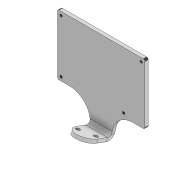
# Autodesk Inventor part: HMI achterzijde
Saved by Autodesk Inventor 2020.3 (Build 243373000, 373)
## iProperties
Created: 2020-12-03
Part Number: HMI achterzijde
Material: Generic
Document SubType Name: Sheet Metal
Designer: Svend
Density: 1 g/cm^3
Sheet Metal Rule: Default_mm
Appearance: Default
Flat Pattern Width: 13.0658 cm
Flat Pattern Length: 10.4848 cm
Flat Pattern Area: 136.992 cm^2
Sheet Metal Width: 130,658 mm
Sheet Metal Length: 104,848 mm
Sheet Metal Area: 13699,236 mm^2
Author: Svend
Autodesk Inventor part; units mm, degrees
ref_plane "YZ Plane" through (0, 0, 0) normal (1, 0, 0) x (0, 1, 0)
ref_plane "XZ Plane" through (0, 0, 0) normal (0, 1, 0) x (-1, 0, 0)
ref_plane "XY Plane" through (0, 0, 0) normal (0, 0, 1) x (1, 0, 0)
ref_plane "Work Plane1" through (0, 0, 0) normal (0, 0, 1) x (1, 0, 0)
sketch "Sketch1" plane through (0, 0, 0) normal (0, 0, 1) x (1, 0, 0)
  line L0 (-22.2591, 4.439) -> (-22.2701, 4.6145)
  line L1 (-22.2701, 4.2636) -> (-22.2591, 4.439)
  line L2 (-22.2701, 4.2636) -> (-22.3031, 4.0909)
  line L3 (-22.3574, 3.9237) -> (-22.3031, 4.0909)
  line L4 (-22.4322, 3.7646) -> (-22.3574, 3.9237)
  line L5 (-22.5265, 3.6161) -> (-22.4322, 3.7646)
  line L6 (-22.6385, 3.4807) -> (-22.5265, 3.6161)
  line L7 (-22.7667, 3.3603) -> (-22.6385, 3.4807)
  line L8 (-22.9089, 3.257) -> (-22.7667, 3.3603)
  line L9 (-23.063, 3.1723) -> (-22.9089, 3.257)
  line L10 (-23.2265, 3.1076) -> (-23.063, 3.1723)
  line L11 (-23.3967, 3.0638) -> (-23.2265, 3.1076)
  line L12 (-23.5712, 3.0418) -> (-23.3967, 3.0638)
  line L13 (-23.747, 3.0418) -> (-23.5712, 3.0418)
  line L14 (-23.9214, 3.0638) -> (-23.747, 3.0418)
  line L15 (-24.0917, 3.1076) -> (-23.9214, 3.0638)
  line L16 (-24.2552, 3.1723) -> (-24.0917, 3.1076)
  line L17 (-24.4092, 3.257) -> (-24.2552, 3.1723)
  line L18 (-24.5515, 3.3603) -> (-24.4092, 3.257)
  line L19 (-24.6796, 3.4807) -> (-24.5515, 3.3603)
  line L20 (-24.7917, 3.6161) -> (-24.6796, 3.4807)
  line L21 (-24.8859, 3.7646) -> (-24.7917, 3.6161)
  line L22 (-24.9608, 3.9237) -> (-24.8859, 3.7646)
  line L23 (-25.0151, 4.0909) -> (-24.9608, 3.9237)
  line L24 (-25.048, 4.2636) -> (-25.0151, 4.0909)
  line L25 (-25.0591, 4.439) -> (-25.048, 4.2636)
  line L26 (-25.048, 4.6145) -> (-25.0591, 4.439)
  line L27 (-25.0151, 4.7872) -> (-25.048, 4.6145)
  line L28 (-24.9608, 4.9544) -> (-25.0151, 4.7872)
  line L29 (-24.8859, 5.1135) -> (-24.9608, 4.9544)
  line L30 (-24.7917, 5.2619) -> (-24.8859, 5.1135)
  line L31 (-24.6796, 5.3974) -> (-24.7917, 5.2619)
  line L32 (-24.5515, 5.5178) -> (-24.6796, 5.3974)
  line L33 (-24.4092, 5.6211) -> (-24.5515, 5.5178)
  line L34 (-24.2552, 5.7058) -> (-24.4092, 5.6211)
  line L35 (-24.0917, 5.7705) -> (-24.2552, 5.7058)
  line L36 (-23.9214, 5.8142) -> (-24.0917, 5.7705)
  line L37 (-23.747, 5.8363) -> (-23.9214, 5.8142)
  line L38 (-23.5712, 5.8363) -> (-23.747, 5.8363)
  line L39 (-23.3967, 5.8142) -> (-23.5712, 5.8363)
  line L40 (-23.2265, 5.7705) -> (-23.3967, 5.8142)
  line L41 (-23.063, 5.7058) -> (-23.2265, 5.7705)
  line L42 (-22.9089, 5.6211) -> (-23.063, 5.7058)
  line L43 (-22.7667, 5.5178) -> (-22.9089, 5.6211)
  line L44 (-22.6385, 5.3974) -> (-22.7667, 5.5178)
  line L45 (-22.5265, 5.2619) -> (-22.6385, 5.3974)
  line L46 (-22.4322, 5.1135) -> (-22.5265, 5.2619)
  line L47 (-22.3574, 4.9544) -> (-22.4322, 5.1135)
  line L48 (-22.3031, 4.7872) -> (-22.3574, 4.9544)
  line L49 (-22.2701, 4.6145) -> (-22.3031, 4.7872)
  line L50 (-1.2701, 68.1645) -> (-1.3031, 68.3372)
  line L51 (-1.2591, 67.989) -> (-1.2701, 68.1645)
  line L52 (-1.2701, 67.8135) -> (-1.2591, 67.989)
  line L53 (-1.2701, 67.8135) -> (-1.3031, 67.6408)
  line L54 (-1.3574, 67.4736) -> (-1.3031, 67.6408)
  line L55 (-1.4323, 67.3145) -> (-1.3574, 67.4736)
  line L56 (-1.5265, 67.1661) -> (-1.4323, 67.3145)
  line L57 (-1.6385, 67.0306) -> (-1.5265, 67.1661)
  line L58 (-1.7667, 66.9103) -> (-1.6385, 67.0306)
  line L59 (-1.9089, 66.8069) -> (-1.7667, 66.9103)
  line L60 (-2.063, 66.7222) -> (-1.9089, 66.8069)
  line L61 (-2.2265, 66.6576) -> (-2.063, 66.7222)
  line L62 (-2.3967, 66.6138) -> (-2.2265, 66.6576)
  line L63 (-2.5712, 66.5918) -> (-2.3967, 66.6138)
  line L64 (-2.747, 66.5918) -> (-2.5712, 66.5918)
  line L65 (-2.9214, 66.6138) -> (-2.747, 66.5918)
  line L66 (-3.0917, 66.6576) -> (-2.9214, 66.6138)
  line L67 (-3.2552, 66.7222) -> (-3.0917, 66.6576)
  line L68 (-3.4092, 66.8069) -> (-3.2552, 66.7222)
  line L69 (-3.5515, 66.9103) -> (-3.4092, 66.8069)
  line L70 (-3.6796, 67.0306) -> (-3.5515, 66.9103)
  line L71 (-3.7917, 67.1661) -> (-3.6796, 67.0306)
  line L72 (-3.8859, 67.3145) -> (-3.7917, 67.1661)
  line L73 (-3.9608, 67.4736) -> (-3.8859, 67.3145)
  line L74 (-4.0151, 67.6408) -> (-3.9608, 67.4736)
  line L75 (-4.048, 67.8135) -> (-4.0151, 67.6408)
  line L76 (-4.0591, 67.989) -> (-4.048, 67.8135)
  line L77 (-4.048, 68.1645) -> (-4.0591, 67.989)
  line L78 (-4.0151, 68.3372) -> (-4.048, 68.1645)
  line L79 (-3.9608, 68.5044) -> (-4.0151, 68.3372)
  line L80 (-3.8859, 68.6635) -> (-3.9608, 68.5044)
  line L81 (-3.7917, 68.8119) -> (-3.8859, 68.6635)
  line L82 (-3.6796, 68.9474) -> (-3.7917, 68.8119)
  line L83 (-3.5515, 69.0677) -> (-3.6796, 68.9474)
  line L84 (-3.4092, 69.1711) -> (-3.5515, 69.0677)
  line L85 (-3.2552, 69.2558) -> (-3.4092, 69.1711)
  line L86 (-3.0917, 69.3205) -> (-3.2552, 69.2558)
  line L87 (-2.9214, 69.3642) -> (-3.0917, 69.3205)
  line L88 (-2.747, 69.3862) -> (-2.9214, 69.3642)
  line L89 (-2.5712, 69.3862) -> (-2.747, 69.3862)
  line L90 (-2.3967, 69.3642) -> (-2.5712, 69.3862)
  line L91 (-2.2265, 69.3205) -> (-2.3967, 69.3642)
  line L92 (-2.063, 69.2558) -> (-2.2265, 69.3205)
  line L93 (-1.9089, 69.1711) -> (-2.063, 69.2558)
  line L94 (-1.7667, 69.0677) -> (-1.9089, 69.1711)
  line L95 (-1.6385, 68.9474) -> (-1.7667, 69.0677)
  line L96 (-1.5265, 68.8119) -> (-1.6385, 68.9474)
  line L97 (-1.4323, 68.6635) -> (-1.5265, 68.8119)
  line L98 (-1.3574, 68.5044) -> (-1.4323, 68.6635)
  line L99 (-1.3031, 68.3372) -> (-1.3574, 68.5044)
  line L100 (-99.0397, 69.3205) -> (-99.2032, 69.2558)
  line L101 (-98.8694, 69.3642) -> (-99.0397, 69.3205)
  line L102 (-98.695, 69.3862) -> (-98.8694, 69.3642)
  line L103 (-98.5192, 69.3862) -> (-98.695, 69.3862)
  line L104 (-98.3448, 69.3642) -> (-98.5192, 69.3862)
  line L105 (-98.1745, 69.3205) -> (-98.3448, 69.3642)
  line L106 (-98.011, 69.2558) -> (-98.1745, 69.3205)
  line L107 (-97.8569, 69.1711) -> (-98.011, 69.2558)
  line L108 (-97.7147, 69.0677) -> (-97.8569, 69.1711)
  line L109 (-97.5865, 68.9474) -> (-97.7147, 69.0677)
  line L110 (-97.4745, 68.8119) -> (-97.5865, 68.9474)
  line L111 (-97.3803, 68.6635) -> (-97.4745, 68.8119)
  line L112 (-97.3054, 68.5044) -> (-97.3803, 68.6635)
  line L113 (-97.2511, 68.3372) -> (-97.3054, 68.5044)
  line L114 (-97.2181, 68.1645) -> (-97.2511, 68.3372)
  line L115 (-97.2071, 67.989) -> (-97.2181, 68.1645)
  line L116 (-97.2181, 67.8135) -> (-97.2071, 67.989)
  line L117 (-97.2181, 67.8135) -> (-97.2511, 67.6408)
  line L118 (-97.3054, 67.4736) -> (-97.2511, 67.6408)
  line L119 (-97.3803, 67.3145) -> (-97.3054, 67.4736)
  line L120 (-97.4745, 67.1661) -> (-97.3803, 67.3145)
  line L121 (-97.5865, 67.0306) -> (-97.4745, 67.1661)
  line L122 (-97.7147, 66.9103) -> (-97.5865, 67.0306)
  line L123 (-97.8569, 66.8069) -> (-97.7147, 66.9103)
  line L124 (-98.011, 66.7222) -> (-97.8569, 66.8069)
  line L125 (-98.1745, 66.6576) -> (-98.011, 66.7222)
  line L126 (-98.3448, 66.6138) -> (-98.1745, 66.6576)
  line L127 (-98.5192, 66.5918) -> (-98.3448, 66.6138)
  line L128 (-98.695, 66.5918) -> (-98.5192, 66.5918)
  line L129 (-98.8694, 66.6138) -> (-98.695, 66.5918)
  line L130 (-99.0397, 66.6576) -> (-98.8694, 66.6138)
  line L131 (-99.2032, 66.7222) -> (-99.0397, 66.6576)
  line L132 (-99.3573, 66.8069) -> (-99.2032, 66.7222)
  line L133 (-99.4995, 66.9103) -> (-99.3573, 66.8069)
  line L134 (-99.6277, 67.0306) -> (-99.4995, 66.9103)
  line L135 (-99.7397, 67.1661) -> (-99.6277, 67.0306)
  line L136 (-99.8339, 67.3145) -> (-99.7397, 67.1661)
  line L137 (-99.9088, 67.4736) -> (-99.8339, 67.3145)
  line L138 (-99.9631, 67.6408) -> (-99.9088, 67.4736)
  line L139 (-99.9961, 67.8135) -> (-99.9631, 67.6408)
  line L140 (-100.0071, 67.989) -> (-99.9961, 67.8135)
  line L141 (-99.9961, 68.1645) -> (-100.0071, 67.989)
  line L142 (-99.9631, 68.3372) -> (-99.9961, 68.1645)
  line L143 (-99.9088, 68.5044) -> (-99.9631, 68.3372)
  line L144 (-99.8339, 68.6635) -> (-99.9088, 68.5044)
  line L145 (-99.7397, 68.8119) -> (-99.8339, 68.6635)
  line L146 (-99.6277, 68.9474) -> (-99.7397, 68.8119)
  line L147 (-99.4995, 69.0677) -> (-99.6277, 68.9474)
  line L148 (-99.3573, 69.1711) -> (-99.4995, 69.0677)
  line L149 (-99.2032, 69.2558) -> (-99.3573, 69.1711)
  line L150 (-99.3573, 3.257) -> (-99.2032, 3.1723)
  line L151 (-99.4995, 3.3603) -> (-99.3573, 3.257)
  line L152 (-99.6277, 3.4807) -> (-99.4995, 3.3603)
  line L153 (-99.7397, 3.6161) -> (-99.6277, 3.4807)
  line L154 (-99.8339, 3.7646) -> (-99.7397, 3.6161)
  line L155 (-99.9088, 3.9237) -> (-99.8339, 3.7646)
  line L156 (-99.9631, 4.0909) -> (-99.9088, 3.9237)
  line L157 (-99.9961, 4.2636) -> (-99.9631, 4.0909)
  line L158 (-100.0071, 4.439) -> (-99.9961, 4.2636)
  line L159 (-99.9961, 4.6145) -> (-100.0071, 4.439)
  line L160 (-99.9631, 4.7872) -> (-99.9961, 4.6145)
  line L161 (-99.9088, 4.9544) -> (-99.9631, 4.7872)
  line L162 (-99.8339, 5.1135) -> (-99.9088, 4.9544)
  line L163 (-99.7397, 5.2619) -> (-99.8339, 5.1135)
  line L164 (-99.6277, 5.3974) -> (-99.7397, 5.2619)
  line L165 (-99.4995, 5.5178) -> (-99.6277, 5.3974)
  line L166 (-99.3573, 5.6211) -> (-99.4995, 5.5178)
  line L167 (-99.2032, 5.7058) -> (-99.3573, 5.6211)
  line L168 (-99.0397, 5.7705) -> (-99.2032, 5.7058)
  line L169 (-98.8694, 5.8142) -> (-99.0397, 5.7705)
  line L170 (-98.695, 5.8363) -> (-98.8694, 5.8142)
  line L171 (-98.5192, 5.8363) -> (-98.695, 5.8363)
  line L172 (-98.3448, 5.8142) -> (-98.5192, 5.8363)
  line L173 (-98.1745, 5.7705) -> (-98.3448, 5.8142)
  line L174 (-98.011, 5.7058) -> (-98.1745, 5.7705)
  line L175 (-97.8569, 5.6211) -> (-98.011, 5.7058)
  line L176 (-97.7147, 5.5178) -> (-97.8569, 5.6211)
  line L177 (-97.5865, 5.3974) -> (-97.7147, 5.5178)
  line L178 (-97.4745, 5.2619) -> (-97.5865, 5.3974)
  line L179 (-97.3803, 5.1135) -> (-97.4745, 5.2619)
  line L180 (-97.3054, 4.9544) -> (-97.3803, 5.1135)
  line L181 (-97.2511, 4.7872) -> (-97.3054, 4.9544)
  line L182 (-97.2181, 4.6145) -> (-97.2511, 4.7872)
  line L183 (-97.2071, 4.439) -> (-97.2181, 4.6145)
  line L184 (-97.2181, 4.2636) -> (-97.2071, 4.439)
  line L185 (-97.2181, 4.2636) -> (-97.2511, 4.0909)
  line L186 (-97.3054, 3.9237) -> (-97.2511, 4.0909)
  line L187 (-97.3803, 3.7646) -> (-97.3054, 3.9237)
  line L188 (-97.4745, 3.6161) -> (-97.3803, 3.7646)
  line L189 (-97.5865, 3.4807) -> (-97.4745, 3.6161)
  line L190 (-97.7147, 3.3603) -> (-97.5865, 3.4807)
  line L191 (-97.8569, 3.257) -> (-97.7147, 3.3603)
  line L192 (-98.011, 3.1723) -> (-97.8569, 3.257)
  line L193 (-98.1745, 3.1076) -> (-98.011, 3.1723)
  line L194 (-98.3448, 3.0638) -> (-98.1745, 3.1076)
  line L195 (-98.5192, 3.0418) -> (-98.3448, 3.0638)
  line L196 (-98.695, 3.0418) -> (-98.5192, 3.0418)
  line L197 (-98.8694, 3.0638) -> (-98.695, 3.0418)
  line L198 (-99.0397, 3.1076) -> (-98.8694, 3.0638)
  line L199 (-99.2032, 3.1723) -> (-99.0397, 3.1076)
  line L200 (0, 0) -> (0.2068, 0.0327)
  line L201 (0.2068, 0.0327) -> (0.409, 0.0869)
  line L202 (0.409, 0.0869) -> (0.6044, 0.162)
  line L203 (0.6044, 0.162) -> (0.7909, 0.257)
  line L204 (0.9665, 0.371) -> (0.7909, 0.257)
  line L205 (0.9665, 0.371) -> (1.1292, 0.5028)
  line L206 (1.1292, 0.5028) -> (1.2772, 0.6508)
  line L207 (1.2772, 0.6508) -> (1.409, 0.8135)
  line L208 (1.409, 0.8135) -> (1.523, 0.989)
  line L209 (1.523, 0.989) -> (1.618, 1.1756)
  line L210 (1.618, 1.1756) -> (1.6931, 1.371)
  line L211 (1.6931, 1.371) -> (1.7472, 1.5732)
  line L212 (1.7472, 1.5732) -> (1.78, 1.78)
  line L213 (1.78, 1.78) -> (1.7909, 1.989)
  line L214 (1.7909, 1.989) -> (1.7909, 5.8277)
  line L215 (1.7909, 5.8277) -> (-0.6591, 5.8277)
  line L216 (-0.6591, 2.439) -> (-0.6591, 5.8277)
  line L217 (-20.6591, 2.439) -> (-0.6591, 2.439)
  line L218 (-20.6591, 2.439) -> (-20.6591, 7.439)
  line L219 (-26.6591, 7.439) -> (-20.6591, 7.439)
  line L220 (-26.6591, 2.439) -> (-26.6591, 7.439)
  line L221 (-26.6591, 2.439) -> (-61.1331, 2.439)
  line L222 (-95.6071, 2.439) -> (-61.1331, 2.439)
  line L223 (-95.6071, 2.439) -> (-95.6071, 7.439)
  line L224 (-100.6071, 7.439) -> (-95.6071, 7.439)
  line L225 (-100.6071, 7.439) -> (-100.6071, 64.989)
  line L226 (-95.6071, 64.989) -> (-100.6071, 64.989)
  line L227 (-95.6071, 69.989) -> (-95.6071, 64.989)
  line L228 (-5.6591, 69.989) -> (-95.6071, 69.989)
  line L229 (-5.6591, 69.989) -> (-5.6591, 64.989)
  line L230 (-5.6591, 64.989) -> (-0.6591, 64.989)
  line L231 (-0.6591, 64.989) -> (-0.6591, 59.8276)
  line L232 (-0.6591, 59.8276) -> (1.7909, 59.8276)
  line L233 (1.7909, 70.439) -> (1.7909, 59.8276)
  line L234 (1.7909, 70.439) -> (1.78, 70.6481)
  line L235 (1.7472, 70.8548) -> (1.78, 70.6481)
  line L236 (1.6931, 71.057) -> (1.7472, 70.8548)
  line L237 (1.618, 71.2525) -> (1.6931, 71.057)
  line L238 (1.618, 71.2525) -> (1.523, 71.439)
  line L239 (1.523, 71.439) -> (1.409, 71.6146)
  line L240 (1.409, 71.6146) -> (1.2772, 71.7773)
  line L241 (1.2772, 71.7773) -> (1.1292, 71.9253)
  line L242 (1.1292, 71.9253) -> (0.9665, 72.057)
  line L243 (0.9665, 72.057) -> (0.7909, 72.1711)
  line L244 (0.7909, 72.1711) -> (0.6044, 72.2661)
  line L245 (0.6044, 72.2661) -> (0.409, 72.3411)
  line L246 (0.409, 72.3411) -> (0.2068, 72.3953)
  line L247 (0.2068, 72.3953) -> (0, 72.428)
  line L248 (-0.2091, 72.439) -> (0, 72.428)
  line L249 (-0.2091, 72.439) -> (-101.0571, 72.439)
  line L250 (-101.0571, 72.439) -> (-101.2661, 72.428)
  line L251 (-101.2661, 72.428) -> (-101.4729, 72.3953)
  line L252 (-101.4729, 72.3953) -> (-101.6751, 72.3411)
  line L253 (-101.6751, 72.3411) -> (-101.8706, 72.2661)
  line L254 (-101.8706, 72.2661) -> (-102.0571, 72.1711)
  line L255 (-102.0571, 72.1711) -> (-102.2327, 72.057)
  line L256 (-102.2327, 72.057) -> (-102.3954, 71.9253)
  line L257 (-102.3954, 71.9253) -> (-102.5434, 71.7773)
  line L258 (-102.5434, 71.7773) -> (-102.6751, 71.6146)
  line L259 (-102.6751, 71.6146) -> (-102.7891, 71.439)
  line L260 (-102.8842, 71.2525) -> (-102.7891, 71.439)
  line L261 (-102.8842, 71.2525) -> (-102.9592, 71.057)
  line L262 (-102.9592, 71.057) -> (-103.0134, 70.8548)
  line L263 (-103.0134, 70.8548) -> (-103.0461, 70.6481)
  line L264 (-103.0571, 70.439) -> (-103.0461, 70.6481)
  line L265 (-103.0571, 1.989) -> (-103.0571, 70.439)
  line L266 (-103.0571, 1.989) -> (-103.0461, 1.78)
  line L267 (-103.0461, 1.78) -> (-103.0134, 1.5732)
  line L268 (-103.0134, 1.5732) -> (-102.9592, 1.371)
  line L269 (-102.8842, 1.1756) -> (-102.9592, 1.371)
  line L270 (-102.8842, 1.1756) -> (-102.7891, 0.989)
  line L271 (-102.7891, 0.989) -> (-102.6751, 0.8135)
  line L272 (-102.6751, 0.8135) -> (-102.5434, 0.6508)
  line L273 (-102.5434, 0.6508) -> (-102.3954, 0.5028)
  line L274 (-102.3954, 0.5028) -> (-102.2327, 0.371)
  line L275 (-102.2327, 0.371) -> (-102.0571, 0.257)
  line L276 (-102.0571, 0.257) -> (-101.8706, 0.162)
  line L277 (-101.8706, 0.162) -> (-101.6751, 0.0869)
  line L278 (-101.6751, 0.0869) -> (-101.4729, 0.0327)
  line L279 (-101.4729, 0.0327) -> (-101.2661, 0)
  line L280 (-101.0571, -0.011) -> (-101.2661, 0)
  line L281 (-101.0571, -0.011) -> (-0.2091, -0.011)
  line L282 (-0.2091, -0.011) -> (0, 0)
  line L283 (1.7909, 5.8277) -> (1.7909, 59.8276)
  line L284 (-103.0571, 1.989) -> (-37.6331, 1.989)
  line L285 (-37.6331, 1.989) -> (-37.6331, -33.011)
  line L286 (-37.6331, -33.011) -> (-63.6331, -33.011)
  line L287 (-63.6331, -33.011) -> (-63.6331, 1.989)
  point P0 (-50.6331, -33.011)
  point P1 (-50.6331, -0.011)
  dimension "d0" = 35
  dimension "d12" = 26
  measures "d0" distance of L284.end L285.end
  measures "d12" distance of L285.end L286.end
extrude "Plate1" add sketch "Sketch1" along normal blind 4
sketch "Sketch2" plane through (-37.6331, -29.2522, -1.3681) normal (0, -0.9396926, 0.3420201) x (1, 0, 0)
  line L0 (-26, 0) -> (0, 0)
  line L1 (0, 0) -> (0, 37)
  line L2 (0, 37) -> (-26, 37)
  line L3 (-26, 37) -> (-26, 0)
  constraints: 6 end point, 1 horizontal, 1 perpendicular, 1 vertical
edge flange "Flange1" height 37 angle 110 thickness 4 bend radius 4 thickness toward (0, -0.9396926, 0.3420201) relief straight relief width 4 relief depth 2 edges at (-50.6331, -33.011, 4) wall of the first edge with corners at (-63.6331, -29.2522, -1.3681) (-37.6331, -29.2522, -1.3681) (-37.6331, -16.5974, 33.4005) (-63.6331, -16.5974, 33.4005)
bend "Bend1"
corner "Corner1"
fillet "Corner Round1" radius 25 2 edges at (-63.6331, -0.011, 2) (-37.6331, -0.011, 2)
fillet "Corner Round2" radius 13 2 edges at (-63.6331, -18.4768, 34.0846) (-37.6331, -18.4768, 34.0846)
sketch "Sketch4" plane through (-63.6331, -25.3445, 9.3681) normal (0, 0.9396926, -0.3420201) x (1, 0, 0)
  circle A0 centre (5.0126, -15.482) radius 2.5 projected
  circle A1 centre (20.9874, -9.6676) radius 2.5 projected
  point P0 (63.6331, 0.1348)
extrude "Cut2" cut sketch "Sketch4" against normal blind 4
equation "\"d17\" = Thickness"
equation "\"d1\" = Thickness"
equation "\"d2\" = BendReliefWidth"
equation "\"d3\" = BendReliefDepth"
equation "\"d4\" = MinimumRemnant"
equation "\"d5\" = TransitionRadius"
equation "\"d8\" = BendRadius"
equation "\"d9\" = CornerReliefSize"
equation "\"d10\" = GapSize"
equation "\"d11\" = JacobiRadiusSize"
equation "\"BendRadius\" = Thickness"
equation "\"BendReliefWidth\" = Thickness"
equation "\"BendReliefDepth\" = 0.5 * Thickness"
equation "\"CornerReliefSize\" = 4 * Thickness"
equation "\"MinimumRemnant\" = 2 * Thickness"
equation "\"TransitionRadius\" = BendRadius"
equation "\"JacobiRadiusSize\" = BendRadius"
equation "\"GapSize\" = Thickness"
equation "\"Thickness\" = 4"
body "Solid1"
